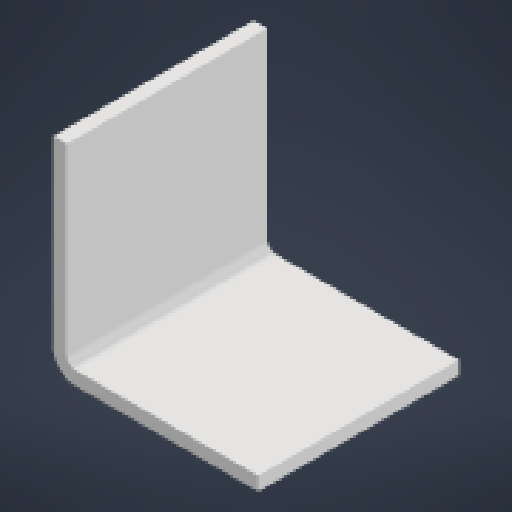
# Autodesk Inventor part: Angle_motor
Saved by Autodesk Inventor 2023.4 (Build 274418000, 418)
## iProperties
Created: 2025-09-23
Part Number: Angle_motor
Material: Generic
Document SubType Name: Modeling
Designer: Malthe Sennels
Density: 1 g/cm^3
Appearance: Default
Author: Malthe Sennels
Autodesk Inventor part; units mm, degrees
ref_plane "YZ Plane" through (0, 0, 0) normal (1, 0, 0) x (0, 1, 0)
ref_plane "XZ Plane" through (0, 0, 0) normal (0, 1, 0) x (-1, 0, 0)
ref_plane "XY Plane" through (0, 0, 0) normal (0, 0, 1) x (1, 0, 0)
sketch "Sketch1" plane through (0, 0, 0) normal (0, 0, 1) x (1, 0, 0)
  line L0 (19, 0) -> (-21, 0)
  line L1 (-26, 0) -> (-26, -3)
  line L2 (-26, -3) -> (19, -3)
  line L3 (19, -3) -> (19, 0)
  line L4 (-26, -3) -> (-23, -3)
  line L5 (-23, 2) -> (-23, 42)
  line L6 (-23, 42) -> (-26, 42)
  line L7 (-26, 42) -> (-26, -3)
  arc A0 (-23, 2) -> (-21, 0) centre (-21, 2) ccw
  arc A1 (-26, 2) -> (-21, -3) centre (-21, 2) ccw
  point P0 (0, 0)
  point P1 (19, -1.5)
  dimension "d0" = 45
  dimension "d1" = 19
  dimension "d2" = 45
  dimension "d3" = 3
  dimension "d4" = 3
  dimension "d5" = 2
  constraints: 16 end point, 5 point on line, 4 parallel, 4 point on circle, 3 tangent, 2 centre point, 2 horizontal, 2 perpendicular, 1 coincident, 1 midpoint
  measures "d0" distance of L2.end L1.end
  measures "d1" horizontal distance of point (19, -1.5) point (0, 0)
  measures "d2" distance of L5.end L4.end
  measures "d3" distance between parallel lines of L7 L5
  measures "d4" distance between parallel lines of L2 L0
  measures "d5" radius of A0
extrude "Extrusion1" add sketch "Sketch1" along normal mid plane 44 contours L3 L2 A1 L7 L6 L5 A0 L0
body "Solid1"
